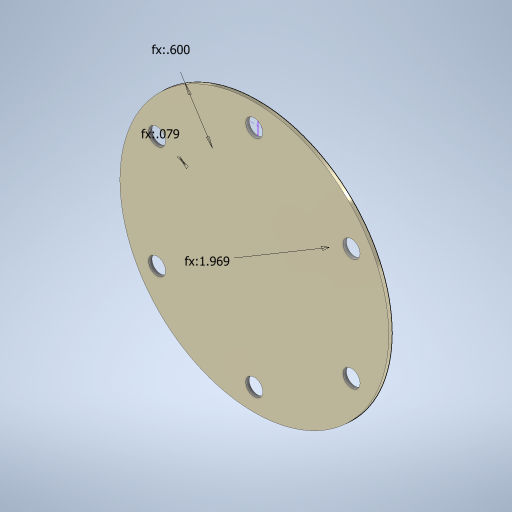
# Autodesk Inventor part: membrane
Saved by Autodesk Inventor 2023 (Build 270158000, 158)
## iProperties
Created: 2023-01-24
Part Number: membrane
Material: Generic
Document SubType Name: Modeling
Designer: remidm
Density: 1 g/cm^3
Appearance: Default
Mass: 0.506707 g
Surface Area: 10.9321 cm^2
Volume: 0.506707 cm^3
MembraneThickness: 0.039 in
Author: remidm
Autodesk Inventor part; units mm, degrees
ref_plane "YZ Plane" through (0, 0, 0) normal (1, 0, 0) x (0, 1, 0)
ref_plane "XZ Plane" through (0, 0, 0) normal (0, 1, 0) x (-1, 0, 0)
ref_plane "XY Plane" through (0, 0, 0) normal (0, 0, 1) x (1, 0, 0)
sketch "Sketch1" plane through (0, 0, 0) normal (0, 0, 1) x (1, 0, 0)
  circle A0 centre (0, 0) radius 40.24
  circle A1 centre (0, 0) radius 25
  circle A2 centre (0, 0) radius 27
  line L0 (0, 33.62) -> (0, 27)
  line L1 (0, 33.62) -> (0, 40.24)
  dimension "d5" = 50
  dimension "d6" = 15.24
  dimension "d17" = 2
  constraints: 4 end point, 3 coincident, 2 vertical alignment, 1 centre point, 1 collinear, 1 point on line, 1 vertical, 4 other
  measures "d5" diameter of A1
extrude "Extrusion1" add sketch "Sketch1" along normal blind 1 contours A0 | A1 | A2
hole "Hole2" at (0, 33.62, 0) direction (0, 0, 1) diameter 5.08 end through all
pattern_circular "Circular Pattern2" count 6 over 360 about axis through (0, 0, 0) along (0, 0, 1) of "Hole2"
equation "\"d5\" = SaltDiameter"
equation "\"d6\" = fixation_extension_length"
equation "\"d17\" = crucible_thickness"
equation "\"d18\" = fixation_holes_diameter"
equation "\"SaltDiameter\" = 50"
equation "\"fixation_extension_length\" = 15.24"
equation "\"crucible_thickness\" = 2"
equation "\"fixation_holes_diameter\" = 5.08"
body "Solid1"
